Autodesk Inventor part; units mm, degrees
(part 2 of 2)
  line L335 (124.4378, 1.3672) -> (124.3595, 1.3442)
  line L336 (124.3595, 1.3442) -> (124.1632, 1.3476)
  line L337 (124.1632, 1.3476) -> (123.9548, 1.3368)
  line L338 (123.9548, 1.3368) -> (123.7636, 1.3115)
  line L339 (123.7636, 1.3115) -> (123.5905, 1.2733)
  line L340 (123.5905, 1.2733) -> (123.4361, 1.2237)
  line L341 (123.4361, 1.2237) -> (123.3011, 1.164)
  line L342 (123.3011, 1.164) -> (123.1861, 1.0959)
  line L343 (123.1861, 1.0959) -> (123.0914, 1.0209)
  line L344 (123.0914, 1.0209) -> (123.0174, 0.9407)
  line L345 (123.0174, 0.9407) -> (122.9644, 0.8567)
  line L346 (122.9644, 0.8567) -> (122.9325, 0.7708)
  line L347 (122.9325, 0.7708) -> (122.9219, 0.6736)
  line L348 (122.9219, 0.6736) -> (122.9381, 0.4362)
  line L349 (122.9381, 0.4362) -> (122.95, 0)
  line L350 (122.95, 0) -> (122.9381, -0.4362)
  line L351 (122.9381, -0.4362) -> (122.9219, -0.6736)
  line L352 (122.9219, -0.6736) -> (122.9325, -0.7708)
  line L353 (122.9325, -0.7708) -> (122.9644, -0.8567)
  line L354 (122.9644, -0.8567) -> (123.0174, -0.9407)
  line L355 (123.0174, -0.9407) -> (123.0914, -1.0209)
  line L356 (123.0914, -1.0209) -> (123.1861, -1.0959)
  line L357 (123.1861, -1.0959) -> (123.3011, -1.164)
  line L358 (123.3011, -1.164) -> (123.4361, -1.2237)
  line L359 (123.4361, -1.2237) -> (123.5905, -1.2733)
  line L360 (123.5905, -1.2733) -> (123.7636, -1.3115)
  line L361 (123.7636, -1.3115) -> (123.9548, -1.3368)
  line L362 (123.9548, -1.3368) -> (124.1632, -1.3476)
  line L363 (124.1632, -1.3476) -> (124.3595, -1.3442)
  line L364 (124.3595, -1.3442) -> (124.4378, -1.3672)
  line L365 (124.4378, -1.3672) -> (124.595, -1.4263)
  line L366 (124.595, -1.4263) -> (124.8086, -1.5275)
  line L367 (124.8086, -1.5275) -> (125.0686, -1.6785)
  line L368 (125.0686, -1.6785) -> (125.2143, -1.7756)
  line L369 (125.2143, -1.7756) -> (125.3694, -1.8885)
  line L370 (125.3694, -1.8885) -> (125.5322, -2.0178)
  line L371 (125.5322, -2.0178) -> (125.7029, -2.1655)
  line L372 (125.7029, -2.1655) -> (125.8775, -2.33)
  line L373 (125.8775, -2.33) -> (126.0577, -2.5143)
  line L374 (126.0577, -2.5143) -> (126.241, -2.7184)
  line L375 (126.241, -2.7184) -> (126.426, -2.9425)
  line L376 (126.426, -2.9425) -> (126.5804, -3.1453)
  arc A6 (126.2175, -4.2622) -> (126.5804, -3.1453) centre (114.9999, 0) ccw
  line L377 (126.2175, -4.2622) -> (125.9734, -4.3355)
  line L378 (125.9734, -4.3355) -> (125.692, -4.4081)
  line L379 (125.692, -4.4081) -> (125.4237, -4.4654)
  line L380 (125.4237, -4.4654) -> (125.1696, -4.5087)
  line L381 (125.1696, -4.5087) -> (124.9317, -4.539)
  line L382 (124.9317, -4.539) -> (124.7067, -4.5582)
  line L383 (124.7067, -4.5582) -> (124.4991, -4.5671)
  line L384 (124.4991, -4.5671) -> (124.3072, -4.5674)
  line L385 (124.3072, -4.5674) -> (124.1322, -4.5603)
  line L386 (124.1322, -4.5603) -> (123.8332, -4.5296)
  line L387 (123.8332, -4.5296) -> (123.6009, -4.4859)
  line L388 (123.6009, -4.4859) -> (123.439, -4.4413)
  line L389 (123.439, -4.4413) -> (123.3621, -4.414)
  line L390 (123.3621, -4.414) -> (123.2053, -4.2958)
  line L391 (123.2053, -4.2958) -> (123.0303, -4.182)
  line L392 (123.0303, -4.182) -> (122.8608, -4.0901)
  line L393 (122.8608, -4.0901) -> (122.6983, -4.0192)
  line L394 (122.6983, -4.0192) -> (122.5442, -3.9687)
  line L395 (122.5442, -3.9687) -> (122.3999, -3.9376)
  line L396 (122.3999, -3.9376) -> (122.2668, -3.9251)
  line L397 (122.2668, -3.9251) -> (122.1462, -3.9301)
  line L398 (122.1462, -3.9301) -> (122.0392, -3.9515)
  line L399 (122.0392, -3.9515) -> (121.9469, -3.9883)
  line L400 (121.9469, -3.9883) -> (121.8706, -4.0391)
  line L401 (121.8706, -4.0391) -> (121.8049, -4.1114)
  line L402 (121.8049, -4.1114) -> (121.6784, -4.313)
  line L403 (121.6784, -4.313) -> (121.4317, -4.6729)
  line L404 (121.4317, -4.6729) -> (121.1656, -5.0188)
  line L405 (121.1656, -5.0188) -> (121.013, -5.2014)
  line L406 (121.013, -5.2014) -> (120.9645, -5.2862)
  line L407 (120.9645, -5.2862) -> (120.9398, -5.3745)
  line L408 (120.9398, -5.3745) -> (120.9333, -5.4735)
  line L409 (120.9333, -5.4735) -> (120.946, -5.5819)
  line L410 (120.946, -5.5819) -> (120.9785, -5.6982)
  line L411 (120.9785, -5.6982) -> (121.0316, -5.821)
  line L412 (121.0316, -5.821) -> (121.1057, -5.9486)
  line L413 (121.1057, -5.9486) -> (121.2014, -6.0795)
  line L414 (121.2014, -6.0795) -> (121.319, -6.2122)
  line L415 (121.319, -6.2122) -> (121.4588, -6.345)
  line L416 (121.4588, -6.345) -> (121.6211, -6.4763)
  line L417 (121.6211, -6.4763) -> (121.782, -6.5889)
  line L418 (121.782, -6.5889) -> (121.8317, -6.6535)
  line L419 (121.8317, -6.6535) -> (121.9242, -6.7937)
  line L420 (121.9242, -6.7937) -> (122.0375, -7.0011)
  line L421 (122.0375, -7.0011) -> (122.1591, -7.2761)
  line L422 (122.1591, -7.2761) -> (122.2199, -7.4403)
  line L423 (122.2199, -7.4403) -> (122.279, -7.6228)
  line L424 (122.279, -7.6228) -> (122.3346, -7.8231)
  line L425 (122.3346, -7.8231) -> (122.3859, -8.0429)
  line L426 (122.3859, -8.0429) -> (122.4306, -8.2786)
  line L427 (122.4306, -8.2786) -> (122.468, -8.5336)
  line L428 (122.468, -8.5336) -> (122.4964, -8.8065)
  line L429 (122.4964, -8.8065) -> (122.5143, -9.0966)
  line L430 (122.5143, -9.0966) -> (122.52, -9.3514)
  arc A7 (121.5699, -10.0416) -> (122.52, -9.3514) centre (115, 0.0001) ccw
  line L431 (121.5699, -10.0416) -> (121.3293, -9.9575)
  line L432 (121.3293, -9.9575) -> (121.059, -9.8508)
  line L433 (121.059, -9.8508) -> (120.8082, -9.7395)
  line L434 (120.8082, -9.7395) -> (120.5773, -9.6252)
  line L435 (120.5773, -9.6252) -> (120.3669, -9.5098)
  line L436 (120.3669, -9.5098) -> (120.1737, -9.3931)
  line L437 (120.1737, -9.3931) -> (120.0004, -9.2783)
  line L438 (120.0004, -9.2783) -> (119.845, -9.1657)
  line L439 (119.845, -9.1657) -> (119.7077, -9.0571)
  line L440 (119.7077, -9.0571) -> (119.4838, -8.8565)
  line L441 (119.4838, -8.8565) -> (119.3215, -8.6847)
  line L442 (119.3215, -8.6847) -> (119.2167, -8.5534)
  line L443 (119.2167, -8.5534) -> (119.1706, -8.4861)
  line L444 (119.1706, -8.4861) -> (119.1133, -8.2983)
  line L445 (119.1133, -8.2983) -> (119.0385, -8.1034)
  line L446 (119.0385, -8.1034) -> (118.9555, -7.9294)
  line L447 (118.9555, -7.9294) -> (118.8656, -7.7765)
  line L448 (118.8656, -7.7765) -> (118.7707, -7.6451)
  line L449 (118.7707, -7.6451) -> (118.6722, -7.5351)
  line L450 (118.6722, -7.5351) -> (118.5719, -7.4468)
  line L451 (118.5719, -7.4468) -> (118.4713, -7.3799)
  line L452 (118.4713, -7.3799) -> (118.3721, -7.3344)
  line L453 (118.3721, -7.3344) -> (118.276, -7.3099)
  line L454 (118.276, -7.3099) -> (118.1843, -7.3061)
  line L455 (118.1843, -7.3061) -> (118.0887, -7.3261)
  line L456 (118.0887, -7.3261) -> (117.8679, -7.4147)
  line L457 (117.8679, -7.4147) -> (117.4567, -7.5609)
  line L458 (117.4567, -7.5609) -> (117.0381, -7.6843)
  line L459 (117.0381, -7.6843) -> (116.8074, -7.7424)
  line L460 (116.8074, -7.7424) -> (116.7182, -7.7825)
  line L461 (116.7182, -7.7825) -> (116.6463, -7.8394)
  line L462 (116.6463, -7.8394) -> (116.5829, -7.9157)
  line L463 (116.5829, -7.9157) -> (116.5294, -8.0109)
  line L464 (116.5294, -8.0109) -> (116.4874, -8.1241)
  line L465 (116.4874, -8.1241) -> (116.4582, -8.2545)
  line L466 (116.4582, -8.2545) -> (116.4431, -8.4013)
  line L467 (116.4431, -8.4013) -> (116.4436, -8.5635)
  line L468 (116.4436, -8.5635) -> (116.4607, -8.74)
  line L469 (116.4607, -8.74) -> (116.4958, -8.9296)
  line L470 (116.4958, -8.9296) -> (116.5499, -9.1312)
  line L471 (116.5499, -9.1312) -> (116.6139, -9.3168)
  line L472 (116.6139, -9.3168) -> (116.6161, -9.3984)
  line L473 (116.6161, -9.3984) -> (116.6085, -9.5662)
  line L474 (116.6085, -9.5662) -> (116.5783, -9.8006)
  line L475 (116.5783, -9.8006) -> (116.515, -10.0945)
  line L476 (116.515, -10.0945) -> (116.4678, -10.2631)
  line L477 (116.4678, -10.2631) -> (116.4082, -10.4455)
  line L478 (116.4082, -10.4455) -> (116.3356, -10.6402)
  line L479 (116.3356, -10.6402) -> (116.2478, -10.8482)
  line L480 (116.2478, -10.8482) -> (116.1454, -11.0652)
  line L481 (116.1454, -11.0652) -> (116.0258, -11.2934)
  line L482 (116.0258, -11.2934) -> (115.8884, -11.5309)
  line L483 (115.8884, -11.5309) -> (115.7324, -11.7761)
  line L484 (115.7324, -11.7761) -> (115.5872, -11.9856)
  arc A8 (114.4128, -11.9856) -> (115.5872, -11.9856) centre (115, 0.0001) ccw
  line L485 (114.4128, -11.9856) -> (114.2676, -11.7761)
  line L486 (114.2676, -11.7761) -> (114.1116, -11.5309)
  line L487 (114.1116, -11.5309) -> (113.9742, -11.2934)
  line L488 (113.9742, -11.2934) -> (113.8546, -11.0652)
  line L489 (113.8546, -11.0652) -> (113.7522, -10.8482)
  line L490 (113.7522, -10.8482) -> (113.6644, -10.6402)
  line L491 (113.6644, -10.6402) -> (113.5918, -10.4455)
  line L492 (113.5918, -10.4455) -> (113.5322, -10.2631)
  line L493 (113.5322, -10.2631) -> (113.485, -10.0945)
  line L494 (113.485, -10.0945) -> (113.4217, -9.8006)
  line L495 (113.4217, -9.8006) -> (113.3915, -9.5662)
  line L496 (113.3915, -9.5662) -> (113.3839, -9.3984)
  line L497 (113.3839, -9.3984) -> (113.3861, -9.3168)
  line L498 (113.3861, -9.3168) -> (113.4501, -9.1312)
  line L499 (113.4501, -9.1312) -> (113.5042, -8.9296)
  line L500 (113.5042, -8.9296) -> (113.5393, -8.74)
  line L501 (113.5393, -8.74) -> (113.5564, -8.5635)
  line L502 (113.5564, -8.5635) -> (113.5569, -8.4013)
  line L503 (113.5569, -8.4013) -> (113.5418, -8.2545)
  line L504 (113.5418, -8.2545) -> (113.5126, -8.1241)
  line L505 (113.5126, -8.1241) -> (113.4706, -8.0109)
  line L506 (113.4706, -8.0109) -> (113.4171, -7.9157)
  line L507 (113.4171, -7.9157) -> (113.3537, -7.8394)
  line L508 (113.3537, -7.8394) -> (113.2818, -7.7825)
  line L509 (113.2818, -7.7825) -> (113.1926, -7.7424)
  line L510 (113.1926, -7.7424) -> (112.9619, -7.6843)
  line L511 (112.9619, -7.6843) -> (112.5433, -7.5609)
  line L512 (112.5433, -7.5609) -> (112.1321, -7.4147)
  line L513 (112.1321, -7.4147) -> (111.9113, -7.3261)
  line L514 (111.9113, -7.3261) -> (111.8157, -7.3061)
  line L515 (111.8157, -7.3061) -> (111.724, -7.3099)
  line L516 (111.724, -7.3099) -> (111.6279, -7.3344)
  line L517 (111.6279, -7.3344) -> (111.5287, -7.3799)
  line L518 (111.5287, -7.3799) -> (111.4281, -7.4468)
  line L519 (111.4281, -7.4468) -> (111.3278, -7.5351)
  line L520 (111.3278, -7.5351) -> (111.2293, -7.6451)
  line L521 (111.2293, -7.6451) -> (111.1344, -7.7765)
  line L522 (111.1344, -7.7765) -> (111.0445, -7.9294)
  line L523 (111.0445, -7.9294) -> (110.9615, -8.1034)
  line L524 (110.9615, -8.1034) -> (110.8867, -8.2983)
  line L525 (110.8867, -8.2983) -> (110.8294, -8.4861)
  line L526 (110.8294, -8.4861) -> (110.7833, -8.5534)
  line L527 (110.7833, -8.5534) -> (110.6785, -8.6847)
  line L528 (110.6785, -8.6847) -> (110.5162, -8.8565)
  line L529 (110.5162, -8.8565) -> (110.2923, -9.0571)
  line L530 (110.2923, -9.0571) -> (110.155, -9.1657)
  line L531 (110.155, -9.1657) -> (109.9996, -9.2783)
  line L532 (109.9996, -9.2783) -> (109.8263, -9.3931)
  line L533 (109.8263, -9.3931) -> (109.6331, -9.5098)
  line L534 (109.6331, -9.5098) -> (109.4227, -9.6252)
  line L535 (109.4227, -9.6252) -> (109.1918, -9.7395)
  line L536 (109.1918, -9.7395) -> (108.941, -9.8508)
  line L537 (108.941, -9.8508) -> (108.6707, -9.9575)
  line L538 (108.6707, -9.9575) -> (108.4301, -10.0416)
  arc A9 (107.48, -9.3514) -> (108.4301, -10.0416) centre (115, 0.0001) ccw
  line L539 (107.48, -9.3514) -> (107.4857, -9.0966)
  constraints: 1080 end point, 20 point on circle, 10 centre point
extrude "Extrusion1" add sketch "layer0" along normal blind 10
extrude "Extrusion2" cut sketch "0" along normal blind 10
body "Solid1"
